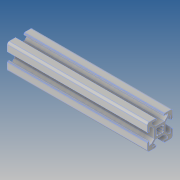
# Autodesk Inventor part: 200-40-BOGIE-CONNECTOR-P-02
Saved by Autodesk Inventor 2018.2 (Build 222227000, 227)
## iProperties
Manager: feesmrt
Company: FRANC0R
Created: 2017-11-20
Part Number: 200-40-BOGIE-CONNECTOR-P-02
Material: Aluminium 6061
Document SubType Name: Modeling
Designer: feesmrt
Density: 2.7 g/cm^3
Appearance: Aluminium - flach
Project: Rescue Robot
Cost Center: -
Description: Bogie Wheel Profile
Engineer: feesmrt
Authority: feesmrt
Stock Number: 200-40-BOGIE-CONNECTOR-P-02
Author: feesmrt
Title: Bogie Wheel Profile
Subject: Rescue Robot
Revision Number: 1
Autodesk Inventor part; units mm, degrees
ref_plane "YZ Plane" through (0, 0, 0) normal (1, 0, 0) x (0, 1, 0)
ref_plane "XZ Plane" through (0, 0, 0) normal (0, 1, 0) x (-1, 0, 0)
ref_plane "XY Plane" through (0, 0, 0) normal (0, 0, 1) x (1, 0, 0)
derived "90-50-PROFILES-20x20xSketch.ipt"
sketch "Skizze2" plane through (0, -3.4393, -4.5) normal (-1, 0, 0) x (0, 0, 1)
  line L0 (10.5, 10.5) -> (10.5, 11.9393)
  line L1 (7.9393, 7.9393) -> (10.5, 10.5)
  line L2 (1.0607, 7.9393) -> (7.9393, 7.9393)
  line L3 (-1.5, 10.5) -> (1.0607, 7.9393)
  line L4 (-1.5, 11.9393) -> (-1.5, 10.5)
  line L5 (1.5, 11.9393) -> (-1.5, 11.9393)
  line L6 (1.5, 12.9393) -> (1.5, 11.9393)
  line L7 (1, 12.9393) -> (1.5, 12.9393)
  line L8 (1, 13.4393) -> (1, 12.9393)
  line L9 (-4, 13.4393) -> (1, 13.4393)
  arc A0 (-4, 13.4393) -> (-5.5, 11.9393) centre (-4, 11.9393) ccw
  line L10 (-5.5, 6.9393) -> (-5.5, 11.9393)
  line L11 (-5, 6.9393) -> (-5.5, 6.9393)
  line L12 (-5, 6.4393) -> (-5, 6.9393)
  line L13 (-4, 6.4393) -> (-5, 6.4393)
  line L14 (-4, 9.4393) -> (-4, 6.4393)
  line L15 (-2.5607, 9.4393) -> (-4, 9.4393)
  line L16 (0, 6.8787) -> (-2.5607, 9.4393)
  line L17 (0, 0) -> (0, 6.8787)
  line L18 (-2.5607, -2.5607) -> (0, 0)
  line L19 (-4, -2.5607) -> (-2.5607, -2.5607)
  line L20 (-4, 0.4393) -> (-4, -2.5607)
  line L21 (-5, 0.4393) -> (-4, 0.4393)
  line L22 (-5, -0.0607) -> (-5, 0.4393)
  line L23 (-5.5, -0.0607) -> (-5, -0.0607)
  line L24 (-5.5, -5.0607) -> (-5.5, -0.0607)
  arc A1 (-5.5, -5.0607) -> (-4, -6.5607) centre (-4, -5.0607) ccw
  line L25 (1, -6.5607) -> (-4, -6.5607)
  line L26 (1, -6.0607) -> (1, -6.5607)
  line L27 (1.5, -6.0607) -> (1, -6.0607)
  line L28 (1.5, -5.0607) -> (1.5, -6.0607)
  line L29 (-1.5, -5.0607) -> (1.5, -5.0607)
  line L30 (-1.5, -3.6213) -> (-1.5, -5.0607)
  line L31 (1.0607, -1.0607) -> (-1.5, -3.6213)
  line L32 (7.9393, -1.0607) -> (1.0607, -1.0607)
  line L33 (10.5, -3.6213) -> (7.9393, -1.0607)
  line L34 (10.5, -5.0607) -> (10.5, -3.6213)
  line L35 (7.5, -5.0607) -> (10.5, -5.0607)
  line L36 (7.5, -6.0607) -> (7.5, -5.0607)
  line L37 (8, -6.0607) -> (7.5, -6.0607)
  line L38 (8, -6.5607) -> (8, -6.0607)
  line L39 (13, -6.5607) -> (8, -6.5607)
  arc A2 (13, -6.5607) -> (14.5, -5.0607) centre (13, -5.0607) ccw
  line L40 (14.5, -0.0607) -> (14.5, -5.0607)
  line L41 (14, -0.0607) -> (14.5, -0.0607)
  line L42 (14, 0.4393) -> (14, -0.0607)
  line L43 (13, 0.4393) -> (14, 0.4393)
  line L44 (13, -2.5607) -> (13, 0.4393)
  line L45 (11.5607, -2.5607) -> (13, -2.5607)
  line L46 (9, 0) -> (11.5607, -2.5607)
  line L47 (9, 6.8787) -> (9, 0)
  line L48 (11.5607, 9.4393) -> (9, 6.8787)
  line L49 (13, 9.4393) -> (11.5607, 9.4393)
  line L50 (13, 6.4393) -> (13, 9.4393)
  line L51 (14, 6.4393) -> (13, 6.4393)
  line L52 (14, 6.9393) -> (14, 6.4393)
  line L53 (14.5, 6.9393) -> (14, 6.9393)
  line L54 (14.5, 11.9393) -> (14.5, 6.9393)
  arc A3 (14.5, 11.9393) -> (13, 13.4393) centre (13, 11.9393) ccw
  line L55 (8, 13.4393) -> (13, 13.4393)
  line L56 (8, 12.9393) -> (8, 13.4393)
  line L57 (7.5, 12.9393) -> (8, 12.9393)
  line L58 (7.5, 11.9393) -> (7.5, 12.9393)
  line L59 (10.5, 11.9393) -> (7.5, 11.9393)
  arc A4 (5.7768, 5.875) -> (3.2232, 5.875) centre (4.5, 3.4393) ccw
  line L60 (5.7768, 5.875) -> (6.4496, 6.4395)
  line L61 (6.4496, 6.4395) -> (7.5002, 5.3889)
  line L62 (7.5002, 5.3889) -> (6.9356, 4.7161)
  arc A5 (6.9356, 2.1626) -> (6.9356, 4.7161) centre (4.5, 3.4393) ccw
  line L63 (6.9356, 2.1626) -> (7.5002, 1.4898)
  line L64 (7.5002, 1.4898) -> (6.4496, 0.4392)
  line L65 (6.4496, 0.4392) -> (5.7768, 1.0037)
  arc A6 (3.2232, 1.0037) -> (5.7768, 1.0037) centre (4.5, 3.4393) ccw
  line L66 (3.2232, 1.0037) -> (2.5504, 0.4392)
  line L67 (2.5504, 0.4392) -> (1.4998, 1.4898)
  line L68 (1.4998, 1.4898) -> (2.0644, 2.1626)
  arc A7 (2.0644, 4.7161) -> (2.0644, 2.1626) centre (4.5, 3.4393) ccw
  line L69 (2.0644, 4.7161) -> (1.4998, 5.3889)
  line L70 (1.4998, 5.3889) -> (2.5504, 6.4395)
  line L71 (2.5504, 6.4395) -> (3.2232, 5.875)
  point P0 (4.5, 3.4393)
extrude "Extrusion3" add sketch "Skizze2" along normal mid plane 110
